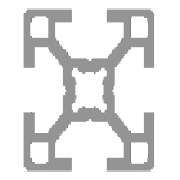
# Autodesk Inventor part: 30-3030
Saved by Autodesk Inventor 2021 (Build 250183000, 183)
## iProperties
_CCFamilyDisplayName: 30-3030
_FrameMemberDoc: Frame Member File
_Version: 25.0.0
_GetPNFromCC: 1
Created: 2020-11-08
Part Number: 30-3030
Material: Generic
Document SubType Name: Modeling
Designer: Wes
Manufacturer: 8020
Standards Organization: 8020 Metric
Language: en-US
Size Designation: 30-3030
Categories: <MemberInstance><Categories><Category DisplayName="Structural Shapes" InternalName="089c4875-fa83-4c05-b084-43b9cc11f5ed" Mnemonic="GRDR"><CategoryParameter DisplayName="Mass per Length Unit" InternalName="0bb95a10-148f-4027-a459-38d7b056702a" Mnemonic="shpmass"/><CategoryParameter DisplayName="Section Area" InternalName="1ff91680-64b0-4202-b9a3-7fd3f94bba3b" Mnemonic="secarea"/><CategoryParameter DisplayName="Radius of Gyration (x)" InternalName="25778675-03e9-40c1-b6a8-4a9ed693320d" Mnemonic="gyrradx"/><CategoryParameter DisplayName="Torsional Rigidity Modulus" InternalName="26c1ec35-5026-4c63-ad0a-751cf684a536" Mnemonic="torrigmod"/><CategoryParameter DisplayName="Distance of the Center of Gravity X-X" InternalName="26c9bdb8-9c79-4b4f-a92e-8e197583c9c4" Mnemonic="grcendistX"/><CategoryParameter DisplayName="Legacy Member ID" InternalName="340afe4f-75d7-48d3-ab7d-943f3c3da468" Mnemonic="LegacyMemberID"/><CategoryParameter DisplayName="Base Length" InternalName="42e34263-8f20-4d0e-ad48-bf1385b87c24" Mnemonic="shplen"/><CategoryParameter DisplayName="Moment of Inertia (y)" InternalName="4b9f58ea-bced-460e-81ea-3d29ca5a49e3" Mnemonic="inermomy"/><CategoryParameter DisplayName="Moment of Inertia (x)" InternalName="4cd780bc-73d7-43ac-917a-579e5cbd684d" Mnemonic="inermomx"/><CategoryParameter DisplayName="Custom Base Point" InternalName="4f1d1b73-316d-484b-a3df-9cbabb16eb77" Mnemonic="shpBasePoint"/><CategoryParameter DisplayName="Shape Height" InternalName="50274e7d-5ac0-4796-92cb-c59e54983c67" Mnemonic="shpheig"/><CategoryParameter DisplayName="Section Module (y)" InternalName="59eaa5e9-d227-48dc-b6c1-6920f96e0f95" Mnemonic="secmody"/><CategoryParameter DisplayName="Section Designation" InternalName="5a64d034-428d-49c8-ba32-7619764de20f" Mnemonic="shpdes"/><CategoryParameter DisplayName="Section Module (x)" InternalName="72cfad18-cf51-4ed4-aaa7-c6b224f8419f" Mnemonic="secmodx"/><CategoryParameter DisplayName="Torsional Section Modulus" InternalName="7c55a8dc-8844-49f9-a867-cc677b30ec9a" Mnemonic="torsecmod"/><CategoryParameter DisplayName="Shape Width" InternalName="7c717d54-a18f-4666-b4d4-573cce22c62c" Mnemonic="shpwdth"/><CategoryParameter DisplayName="Second Shape Thickness" InternalName="9251a8e1-85fd-4e47-af99-afdb762317d9" Mnemonic="shpthick2"/><CategoryParameter DisplayName="FG Authored" InternalName="9c666724-f362-4ea7-ac62-f6a007de5c69" Mnemonic="shpFGAuto"/><CategoryParameter DisplayName="Distance of the Center of Gravity Y-Y" InternalName="bcc4fb17-7af4-436a-8f8c-d0aa3b0248c5" Mnemonic="grcendistY"/><CategoryParameter DisplayName="Radius of Gyration (y)" InternalName="bfa18ebe-1636-4dbe-8d42-b263e0b73184" Mnemonic="gyrrady"/><CategoryParameter DisplayName="Shape Thickness" InternalName="d109cf76-8eb4-42fc-9800-4409734adc67" Mnemonic="shpthick"/><CategoryParameter DisplayName="Coefficient of Shear Displacement" InternalName="de4c90c6-aaa8-468f-a335-6737b311b5d3" Mnemonic="shdispc"/><Category DisplayName="Other" InternalName="f02205ff-2390-476f-921c-0b3185f88e84" Mnemonic="OTHSHP"><CategoryParameter DisplayName="Moment of Inertia (y)" InternalName="044c654e-f649-48ac-84cc-650a29ae31ca" Mnemonic="inermomy"/><CategoryParameter DisplayName="Shape Thickness" InternalName="12b1a788-9233-48fd-a933-2df8ff42b15f" Mnemonic="shpthick"/><CategoryParameter DisplayName="Mass per Length Unit" InternalName="2fd289d6-9394-4d2d-97e6-6659d7d4551d" Mnemonic="shpmass"/><CategoryParameter DisplayName="Radius of Gyration (y)" InternalName="743e1dfe-1bba-408b-b985-cf752b207386" Mnemonic="gyrrady"/><CategoryParameter DisplayName="Section Module (y)" InternalName="88b8bff9-a616-4028-93d5-ed4f79680d13" Mnemonic="secmody"/><CategoryParameter DisplayName="Section Area" InternalName="c46ecdf8-b6eb-4db9-8b25-30258930c1e3" Mnemonic="secarea"/><CategoryParameter DisplayName="Section Module (x)" InternalName="cac70804-9d39-43bb-be17-56ea1f39a6c2" Mnemonic="secmodx"/><CategoryParameter DisplayName="Moment of Inertia (x)" InternalName="ec6737bc-264f-43ed-b0bd-f6d410c2718d" Mnemonic="inermomx"/><CategoryParameter DisplayName="Radius of Gyration (x)" InternalName="ee72c61e-565e-4fd6-b448-66e1e1abcb7e" Mnemonic="gyrradx"/><Category DisplayName="8020" InternalName="79851eee-1260-43d5-80eb-d25638456875" Mnemonic="8020"/></Category></Category><Category DisplayName="DataType" InternalName="23b78d0f-2648-40c6-8793-ca6db495c9e8" Mnemonic="DATATYPE"><CategoryParameter DisplayName="DisplayName" InternalName="05415f3d-3907-474b-a020-eb9d644f4cf3" Mnemonic="DISPLAYNAME"/><CategoryParameter DisplayName="Standard" InternalName="0c0a119c-1e12-4c84-803f-101930972f5e" Mnemonic="STANDARD"/><CategoryParameter DisplayName="Description" InternalName="13903e3d-64b1-4950-80da-f627842ea37f" Mnemonic="DESCRIPTION"/><CategoryParameter DisplayName="Designation" InternalName="2675968c-4ce5-49e0-a4f5-552d29089031" Mnemonic="DESIGNATION"/><CategoryParameter DisplayName="Default Row" InternalName="2af9ec52-faaa-4026-b378-f9fa4afca842" Mnemonic="DEFAULTROW"/><CategoryParameter DisplayName="Folder Name" InternalName="3f06958e-8713-4116-9be7-ed6184ecc97b" Mnemonic="FOLDERNAME"/><CategoryParameter DisplayName="Revision Guid" InternalName="45a75005-10b1-4dfc-8d6d-dfe629f0b93c" Mnemonic="REVISIONGUID"/><CategoryParameter DisplayName="FileName" InternalName="8b46a4cc-9585-4fed-90c3-899f57e09a73" Mnemonic="FILENAME"/><CategoryParameter DisplayName="StdsOrg" InternalName="8f5914e1-4693-403f-8ab5-d37768198c9d" Mnemonic="STDSORG"/><CategoryParameter DisplayName="Family Version" InternalName="914462f6-6e19-4b14-ba84-155b9680b1d0" Mnemonic="FAMILYREVISION"/><CategoryParameter DisplayName="Standard Revision" InternalName="91d5a463-65c2-4fde-b823-3b7fea5e8e17" Mnemonic="STANDARDREVISION"/><CategoryParameter DisplayName="Member Revision" InternalName="a65d44b9-392f-4f4f-857b-e4b3d54996fe" Mnemonic="MEMBERREVISION"/><CategoryParameter DisplayName="ClipFormat" InternalName="bc51e27b-3422-4e78-93ef-cec197ddf230" Mnemonic="CLIPFORMAT"/><CategoryParameter DisplayName="Manufacturer" InternalName="cd6c7a72-a28a-4e50-99a9-2c7f4e13e5ad" Mnemonic="MANUFACTURER"/><CategoryParameter DisplayName="InternalName" InternalName="cf1d0246-76d9-4b4a-8305-fa0409afb5c1" Mnemonic="INTERNALNAME"/><CategoryParameter DisplayName="IsMetric" InternalName="e2385c5b-1ea4-4823-96a8-8de651266ec3" Mnemonic="ISMETRIC"/><Category DisplayName="Part" InternalName="c0e0b642-3bcb-4cc8-9e80-f96d35c4afa4" Mnemonic="PART"><CategoryParameter DisplayName="Part Number" InternalName="016b6077-bfbe-49bd-92c9-d8d59c39c941" Mnemonic="PARTNUMBER"/><CategoryParameter DisplayName="Stock Number" InternalName="4dba7c1c-e26c-444e-836c-b08b433409a8" Mnemonic="STOCKNUMBER"/><CategoryParameter DisplayName="Material Key" InternalName="5c9a8adb-dd2b-4535-b97f-0a94a95fe41f" Mnemonic="MATERIALKEY"/><CategoryParameter DisplayName="Material" InternalName="818a152a-d3c3-49ca-80ee-df7d91421b8e" Mnemonic="MATERIAL"/></Category></Category></Categories><FamilyTemplate Id="30-3030"><FamilyTemplateParameters><FamilyTemplateParameter ObjectType="kModelParameterObject" ValueType="xs:double" Id="12" ObjectReferenceKey="Length"/><FamilyTemplateParameter ObjectType="kPartComponentDefinitionObject" ValueType="xs:string" Id="23" SubObjectId="Material"/><FamilyTemplateParameter ObjectType="kPropertyObject" ValueType="xs:string" Id="26" ObjectReferenceKey="{32853F0F-3444-11d1-9E93-0060B03C1CA6}" SubObjectId="5"/><FamilyTemplateParameter ObjectType="kPropertyObject" ValueType="xs:string" Id="27" ObjectReferenceKey="{32853F0F-3444-11d1-9E93-0060B03C1CA6}" SubObjectId="52"/></FamilyTemplateParameters></FamilyTemplate><CategoryParameterMap><ParamToTemplateMap><ParamToTemplate CategoryParameter="//CategoryParameter[@InternalName='cf1d0246-76d9-4b4a-8305-fa0409afb5c1']" ConstantValue="0c7d1244-42aa-4641-8c1f-ef9d9099bed6"/><ParamToTemplate CategoryParameter="//CategoryParameter[@InternalName='45a75005-10b1-4dfc-8d6d-dfe629f0b93c']" ConstantValue="15f48215-b719-44ce-96ed-f2adf66c00d4"/><ParamToTemplate CategoryParameter="//CategoryParameter[@InternalName='3f06958e-8713-4116-9be7-ed6184ecc97b']" ConstantValue="30-3030"/><ParamToTemplate CategoryParameter="//CategoryParameter[@InternalName='8f5914e1-4693-403f-8ab5-d37768198c9d']" ConstantValue="8020 Metric"/><ParamToTemplate CategoryParameter="//CategoryParameter[@InternalName='0c0a119c-1e12-4c84-803f-101930972f5e']" TemplateParameter="18"/><ParamToTemplate CategoryParameter="//CategoryParameter[@InternalName='91d5a463-65c2-4fde-b823-3b7fea5e8e17']" TemplateParameter="19"/><ParamToTemplate CategoryParameter="//CategoryParameter[@InternalName='cd6c7a72-a28a-4e50-99a9-2c7f4e13e5ad']" ConstantValue="8020"/><ParamToTemplate CategoryParameter="//CategoryParameter[@InternalName='13903e3d-64b1-4950-80da-f627842ea37f']" TemplateParameter="22"/><ParamToTemplate CategoryParameter="//CategoryParameter[@InternalName='05415f3d-3907-474b-a020-eb9d644f4cf3']" ConstantValue="30-3030"/><ParamToTemplate CategoryParameter="//CategoryParameter[@InternalName='914462f6-6e19-4b14-ba84-155b9680b1d0']" ConstantValue="11"/><ParamToTemplate CategoryParameter="//CategoryParameter[@InternalName='bc51e27b-3422-4e78-93ef-cec197ddf230']" ConstantValue="CF_INVENTOR.STDPARTS"/><ParamToTemplate CategoryParameter="//CategoryParameter[@InternalName='e2385c5b-1ea4-4823-96a8-8de651266ec3']" ConstantValue="false"/><ParamToTemplate CategoryParameter="//CategoryParameter[@InternalName='2af9ec52-faaa-4026-b378-f9fa4afca842']" ConstantValue="1"/><ParamToTemplate CategoryParameter="//CategoryParameter[@InternalName='9c666724-f362-4ea7-ac62-f6a007de5c69']" ConstantValue="1"/><ParamToTemplate CategoryParameter="//CategoryParameter[@InternalName='8b46a4cc-9585-4fed-90c3-899f57e09a73']" ConstantValue="30-3030"/><ParamToTemplate CategoryParameter="//CategoryParameter[@InternalName='a65d44b9-392f-4f4f-857b-e4b3d54996fe']" ConstantValue="83db84f2-a349-434c-8932-27b256aad8d1"/><ParamToTemplate CategoryParameter="//CategoryParameter[@InternalName='a65d44b9-392f-4f4f-857b-e4b3d54996fe']" ConstantValue="83db84f2-a349-434c-8932-27b256aad8d1"/><ParamToTemplate CategoryParameter="//CategoryParameter[@InternalName='2675968c-4ce5-49e0-a4f5-552d29089031']" TemplateParameter="27"/><ParamToTemplate CategoryParameter="//CategoryParameter[@InternalName='42e34263-8f20-4d0e-ad48-bf1385b87c24']" TemplateParameter="12"/><ParamToTemplate CategoryParameter="//CategoryParameter[@InternalName='818a152a-d3c3-49ca-80ee-df7d91421b8e']" TemplateParameter="23"/><ParamToTemplate CategoryParameter="//CategoryParameter[@InternalName='016b6077-bfbe-49bd-92c9-d8d59c39c941']" TemplateParameter="26"/></ParamToTemplateMap></CategoryParameterMap></MemberInstance>
Density: 1 g/cm^3
Appearance: Default
IsCustomPart: 1
G_W: 1.181 in
G_H: 1.181 in
G_L: 34.016 in
+F1501FAD-5F95-4806-B732-5FE33EAD4360+CUTDETAIL1: Cut Angle 90.00 deg
Author: Wes
Autodesk Inventor part; units mm, degrees
sketch "30-3030" plane through (0, 0, 0) normal (0, 0, 1) x (1, 0, 0)
  arc A0 (-12.7342, 25.6778) -> (-12.3542, 25.2978) centre (-12.3542, 25.6778) ccw
  line L0 (-12.3542, 25.2978) -> (-8.9152, 25.2978)
  arc A1 (-8.9152, 25.2978) -> (-8.5342, 25.6788) centre (-8.9152, 25.6788) ccw
  line L1 (-8.5342, 25.6788) -> (-8.5342, 28.4978)
  arc A2 (-8.5342, 28.4978) -> (-9.5342, 29.4978) centre (-9.5342, 28.4978) ccw
  line L2 (-9.5342, 29.4978) -> (-12.3532, 29.4978)
  arc A3 (-12.3532, 29.4978) -> (-12.7342, 29.1168) centre (-12.3532, 29.1168) ccw
  line L3 (-12.7342, 29.1168) -> (-12.7342, 25.6778)
  arc A4 (-19.7608, 11.8179) -> (-18.2542, 13.3245) centre (-19.0919, 12.6556) ccw
  line L4 (-18.2542, 13.3245) -> (-19.036, 14.3036)
  arc A5 (-19.036, 14.3036) -> (-19.036, 17.2921) centre (-22.2341, 15.7978) ccw
  line L5 (-19.036, 17.2921) -> (-18.2542, 18.2712)
  arc A6 (-18.2542, 18.2712) -> (-19.7608, 19.7778) centre (-19.0919, 18.94) ccw
  line L6 (-19.7608, 19.7778) -> (-20.7399, 18.996)
  arc A7 (-20.7399, 18.996) -> (-23.7283, 18.996) centre (-22.2341, 15.7978) ccw
  line L7 (-23.7283, 18.996) -> (-24.7075, 19.7778)
  arc A8 (-24.7075, 19.7778) -> (-26.214, 18.2712) centre (-25.3763, 18.94) ccw
  line L8 (-26.214, 18.2712) -> (-25.4323, 17.2921)
  arc A9 (-25.4323, 17.2921) -> (-25.4323, 14.3036) centre (-22.2341, 15.7978) ccw
  line L9 (-25.4323, 14.3036) -> (-26.214, 13.3245)
  arc A10 (-26.214, 13.3245) -> (-24.7075, 11.8179) centre (-25.3763, 12.6556) ccw
  line L10 (-24.7075, 11.8179) -> (-23.7283, 12.5997)
  arc A11 (-23.7283, 12.5997) -> (-20.7399, 12.5997) centre (-22.2341, 15.7978) ccw
  line L11 (-20.7399, 12.5997) -> (-19.7608, 11.8179)
  arc A12 (-9.5342, 2.0979) -> (-8.5342, 3.0979) centre (-9.5342, 3.0979) ccw
  line L12 (-8.5342, 3.0979) -> (-8.5342, 5.9169)
  arc A13 (-8.5342, 5.9169) -> (-8.9152, 6.2979) centre (-8.9152, 5.9169) ccw
  line L13 (-8.9152, 6.2979) -> (-12.3542, 6.2979)
  arc A14 (-12.3542, 6.2979) -> (-12.7342, 5.9179) centre (-12.3542, 5.9179) ccw
  line L14 (-12.7342, 5.9179) -> (-12.7342, 2.4789)
  arc A15 (-12.7342, 2.4789) -> (-12.3532, 2.0979) centre (-12.3532, 2.4789) ccw
  line L15 (-12.3532, 2.0979) -> (-9.5342, 2.0979)
  line L16 (-7.7342, 11.7978) -> (-8.9916, 11.7978)
  arc A16 (-7.2342, 11.2978) -> (-7.7342, 11.7978) centre (-7.7342, 11.2978) ccw
  line L17 (-7.2342, 2.7979) -> (-7.2342, 11.2978)
  arc A17 (-9.2342, 0.7979) -> (-7.2342, 2.7979) centre (-9.2342, 2.7979) ccw
  line L18 (-17.7341, 0.7979) -> (-9.2342, 0.7979)
  arc A18 (-18.2341, 1.2979) -> (-17.7341, 0.7979) centre (-17.7341, 1.2979) ccw
  line L19 (-18.2341, 2.5554) -> (-18.2341, 1.2979)
  arc A19 (-17.7341, 3.0554) -> (-18.2341, 2.5554) centre (-17.7341, 2.5554) ccw
  line L20 (-14.5016, 3.0554) -> (-17.7341, 3.0554)
  arc A20 (-14.5016, 3.0554) -> (-13.9842, 3.555) centre (-14.4841, 3.555) ccw
  line L21 (-13.9842, 5.5376) -> (-13.9842, 3.555)
  arc A21 (-13.9842, 5.5376) -> (-14.1306, 5.8912) centre (-14.4841, 5.5376) ccw
  line L22 (-18.0561, 9.8167) -> (-14.1306, 5.8912)
  arc A22 (-18.0561, 9.8167) -> (-18.4097, 9.9632) centre (-18.4097, 9.4632) ccw
  line L23 (-21.2841, 9.9632) -> (-18.4097, 9.9632)
  line L24 (-22.2341, 10.4732) -> (-21.2841, 9.9632)
  line L25 (-23.1841, 9.9632) -> (-22.2341, 10.4732)
  line L26 (-26.0586, 9.9632) -> (-23.1841, 9.9632)
  arc A23 (-26.0586, 9.9632) -> (-26.4121, 9.8167) centre (-26.0586, 9.4632) ccw
  line L27 (-30.3376, 5.8912) -> (-26.4121, 9.8167)
  arc A24 (-30.3376, 5.8912) -> (-30.4841, 5.5376) centre (-29.9841, 5.5376) ccw
  line L28 (-30.4841, 3.555) -> (-30.4841, 5.5376)
  arc A25 (-30.4841, 3.555) -> (-29.9666, 3.0554) centre (-29.9841, 3.555) ccw
  line L29 (-26.7341, 3.0554) -> (-29.9666, 3.0554)
  arc A26 (-26.2341, 2.5554) -> (-26.7341, 3.0554) centre (-26.7341, 2.5554) ccw
  line L30 (-26.2341, 1.2979) -> (-26.2341, 2.5554)
  arc A27 (-26.7341, 0.7979) -> (-26.2341, 1.2979) centre (-26.7341, 1.2979) ccw
  line L31 (-35.2341, 0.7979) -> (-26.7341, 0.7979)
  arc A28 (-37.2341, 2.7979) -> (-35.2341, 0.7979) centre (-35.2341, 2.7979) ccw
  line L32 (-37.2341, 11.2978) -> (-37.2341, 2.7979)
  arc A29 (-36.7341, 11.7978) -> (-37.2341, 11.2978) centre (-36.7341, 11.2978) ccw
  line L33 (-35.4766, 11.7978) -> (-36.7341, 11.7978)
  arc A30 (-34.9766, 11.2978) -> (-35.4766, 11.7978) centre (-35.4766, 11.2978) ccw
  line L34 (-34.9766, 8.0653) -> (-34.9766, 11.2978)
  arc A31 (-34.9766, 8.0653) -> (-34.4769, 7.5479) centre (-34.4769, 8.0479) ccw
  line L35 (-32.4943, 7.5479) -> (-34.4769, 7.5479)
  arc A32 (-32.4943, 7.5479) -> (-32.1408, 7.6943) centre (-32.4943, 8.0479) ccw
  line L36 (-28.2152, 11.6198) -> (-32.1408, 7.6943)
  arc A33 (-28.2152, 11.6198) -> (-28.0688, 11.9734) centre (-28.5688, 11.9734) ccw
  line L37 (-28.0688, 14.7853) -> (-28.0688, 11.9734)
  line L38 (-27.5588, 15.7353) -> (-28.0688, 14.7853)
  line L39 (-28.0688, 16.6853) -> (-27.5588, 15.7353)
  line L40 (-28.0688, 19.6223) -> (-28.0688, 16.6853)
  arc A34 (-28.0688, 19.6223) -> (-28.2152, 19.9758) centre (-28.5688, 19.6223) ccw
  line L41 (-32.1408, 23.9013) -> (-28.2152, 19.9758)
  arc A35 (-32.1408, 23.9013) -> (-32.4943, 24.0478) centre (-32.4943, 23.5478) ccw
  line L42 (-34.4769, 24.0478) -> (-32.4943, 24.0478)
  arc A36 (-34.4769, 24.0478) -> (-34.9766, 23.5303) centre (-34.4769, 23.5478) ccw
  line L43 (-34.9766, 20.2978) -> (-34.9766, 23.5303)
  arc A37 (-35.4766, 19.7978) -> (-34.9766, 20.2978) centre (-35.4766, 20.2978) ccw
  line L44 (-36.7341, 19.7978) -> (-35.4766, 19.7978)
  arc A38 (-37.2341, 20.2978) -> (-36.7341, 19.7978) centre (-36.7341, 20.2978) ccw
  line L45 (-37.2341, 28.7978) -> (-37.2341, 20.2978)
  arc A39 (-35.2341, 30.7978) -> (-37.2341, 28.7978) centre (-35.2341, 28.7978) ccw
  line L46 (-26.7341, 30.7978) -> (-35.2341, 30.7978)
  arc A40 (-26.2341, 30.2978) -> (-26.7341, 30.7978) centre (-26.7341, 30.2978) ccw
  line L47 (-26.2341, 29.0403) -> (-26.2341, 30.2978)
  arc A41 (-26.7341, 28.5403) -> (-26.2341, 29.0403) centre (-26.7341, 29.0403) ccw
  line L48 (-29.9666, 28.5403) -> (-26.7341, 28.5403)
  arc A42 (-29.9666, 28.5403) -> (-30.4841, 28.0406) centre (-29.9841, 28.0406) ccw
  line L49 (-30.4841, 26.058) -> (-30.4841, 28.0406)
  arc A43 (-30.4841, 26.058) -> (-30.3376, 25.7045) centre (-29.9841, 26.058) ccw
  line L50 (-26.4121, 21.7789) -> (-30.3376, 25.7045)
  arc A44 (-26.4121, 21.7789) -> (-26.0586, 21.6325) centre (-26.0586, 22.1325) ccw
  line L51 (-23.1841, 21.6325) -> (-26.0586, 21.6325)
  line L52 (-22.2341, 21.1225) -> (-23.1841, 21.6325)
  line L53 (-21.2841, 21.6325) -> (-22.2341, 21.1225)
  line L54 (-18.4097, 21.6325) -> (-21.2841, 21.6325)
  arc A45 (-18.4097, 21.6325) -> (-18.0561, 21.7789) centre (-18.4097, 22.1325) ccw
  line L55 (-14.1306, 25.7045) -> (-18.0561, 21.7789)
  arc A46 (-14.1306, 25.7045) -> (-13.9842, 26.058) centre (-14.4841, 26.058) ccw
  line L56 (-13.9842, 28.0406) -> (-13.9842, 26.058)
  arc A47 (-13.9842, 28.0406) -> (-14.5016, 28.5403) centre (-14.4841, 28.0406) ccw
  line L57 (-17.7341, 28.5403) -> (-14.5016, 28.5403)
  arc A48 (-18.2341, 29.0403) -> (-17.7341, 28.5403) centre (-17.7341, 29.0403) ccw
  line L58 (-18.2341, 30.2978) -> (-18.2341, 29.0403)
  arc A49 (-17.7341, 30.7978) -> (-18.2341, 30.2978) centre (-17.7341, 30.2978) ccw
  line L59 (-9.2342, 30.7978) -> (-17.7341, 30.7978)
  arc A50 (-7.2342, 28.7978) -> (-9.2342, 30.7978) centre (-9.2342, 28.7978) ccw
  line L60 (-7.2342, 20.2978) -> (-7.2342, 28.7978)
  arc A51 (-7.7342, 19.7978) -> (-7.2342, 20.2978) centre (-7.7342, 20.2978) ccw
  line L61 (-8.9916, 19.7978) -> (-7.7342, 19.7978)
  arc A52 (-9.4916, 20.2978) -> (-8.9916, 19.7978) centre (-8.9916, 20.2978) ccw
  line L62 (-9.4916, 23.5303) -> (-9.4916, 20.2978)
  arc A53 (-9.4916, 23.5303) -> (-9.9913, 24.0478) centre (-9.9913, 23.5478) ccw
  line L63 (-11.9739, 24.0478) -> (-9.9913, 24.0478)
  arc A54 (-11.9739, 24.0478) -> (-12.3275, 23.9013) centre (-11.9739, 23.5478) ccw
  line L64 (-16.253, 19.9758) -> (-12.3275, 23.9013)
  arc A55 (-16.253, 19.9758) -> (-16.3994, 19.6223) centre (-15.8994, 19.6223) ccw
  line L65 (-16.3994, 16.6853) -> (-16.3994, 19.6223)
  line L66 (-16.9094, 15.7353) -> (-16.3994, 16.6853)
  line L67 (-16.3994, 14.7853) -> (-16.9094, 15.7353)
  line L68 (-16.3994, 11.9734) -> (-16.3994, 14.7853)
  arc A56 (-16.3994, 11.9734) -> (-16.253, 11.6198) centre (-15.8994, 11.9734) ccw
  line L69 (-12.3275, 7.6943) -> (-16.253, 11.6198)
  arc A57 (-12.3275, 7.6943) -> (-11.9739, 7.5479) centre (-11.9739, 8.0479) ccw
  line L70 (-9.9913, 7.5479) -> (-11.9739, 7.5479)
  arc A58 (-9.9913, 7.5479) -> (-9.4916, 8.0653) centre (-9.9913, 8.0479) ccw
  line L71 (-9.4916, 11.2978) -> (-9.4916, 8.0653)
  arc A59 (-8.9916, 11.7978) -> (-9.4916, 11.2978) centre (-8.9916, 11.2978) ccw
  arc A60 (-35.9341, 3.0979) -> (-34.9341, 2.0979) centre (-34.9341, 3.0979) ccw
  line L72 (-34.9341, 2.0979) -> (-32.1151, 2.0979)
  arc A61 (-32.1151, 2.0979) -> (-31.7341, 2.4789) centre (-32.1151, 2.4789) ccw
  line L73 (-31.7341, 2.4789) -> (-31.7341, 5.9179)
  arc A62 (-31.7341, 5.9179) -> (-32.1141, 6.2979) centre (-32.1141, 5.9179) ccw
  line L74 (-32.1141, 6.2979) -> (-35.5531, 6.2979)
  arc A63 (-35.5531, 6.2979) -> (-35.9341, 5.9169) centre (-35.5531, 5.9169) ccw
  line L75 (-35.9341, 5.9169) -> (-35.9341, 3.0979)
  arc A64 (-34.9341, 29.4978) -> (-35.9341, 28.4978) centre (-34.9341, 28.4978) ccw
  line L76 (-35.9341, 28.4978) -> (-35.9341, 25.6788)
  arc A65 (-35.9341, 25.6788) -> (-35.5531, 25.2978) centre (-35.5531, 25.6788) ccw
  line L77 (-35.5531, 25.2978) -> (-32.1141, 25.2978)
  arc A66 (-32.1141, 25.2978) -> (-31.7341, 25.6778) centre (-32.1141, 25.6778) ccw
  line L78 (-31.7341, 25.6778) -> (-31.7341, 29.1168)
  arc A67 (-31.7341, 29.1168) -> (-32.1151, 29.4978) centre (-32.1151, 29.1168) ccw
  line L79 (-32.1151, 29.4978) -> (-34.9341, 29.4978)
ref_plane "Start Plane" through (0, 0, -29.9999) normal (0, 0, 1) x (1, 0, 0)
ref_plane "End Plane" through (0, 0, 834) normal (0, 0, 1) x (1, 0, 0)
sketch "Sketch" plane through (0, 0, 0) normal (0, 0, 1) x (1, 0, 0)
  arc A0 (9.5, 9.88) -> (9.88, 9.5) centre (9.88, 9.88) ccw
  line L0 (9.88, 9.5) -> (13.3189, 9.5)
  arc A1 (13.3189, 9.5) -> (13.6999, 9.881) centre (13.3189, 9.881) ccw
  line L1 (13.6999, 9.881) -> (13.6999, 12.6999)
  arc A2 (13.6999, 12.6999) -> (12.6999, 13.6999) centre (12.6999, 12.6999) ccw
  line L2 (12.6999, 13.6999) -> (9.881, 13.6999)
  arc A3 (9.881, 13.6999) -> (9.5, 13.3189) centre (9.881, 13.3189) ccw
  line L3 (9.5, 13.3189) -> (9.5, 9.88)
  arc A4 (2.4733, -3.9799) -> (3.9799, -2.4733) centre (3.1422, -3.1422) ccw
  line L4 (3.9799, -2.4733) -> (3.1981, -1.4942)
  arc A5 (3.1981, -1.4942) -> (3.1981, 1.4942) centre (0, 0) ccw
  line L5 (3.1981, 1.4942) -> (3.9799, 2.4733)
  arc A6 (3.9799, 2.4733) -> (2.4733, 3.9799) centre (3.1422, 3.1422) ccw
  line L6 (2.4733, 3.9799) -> (1.4942, 3.1981)
  arc A7 (1.4942, 3.1981) -> (-1.4942, 3.1981) centre (0, 0) ccw
  line L7 (-1.4942, 3.1981) -> (-2.4733, 3.9799)
  arc A8 (-2.4733, 3.9799) -> (-3.9799, 2.4733) centre (-3.1422, 3.1422) ccw
  line L8 (-3.9799, 2.4733) -> (-3.1981, 1.4942)
  arc A9 (-3.1981, 1.4942) -> (-3.1981, -1.4942) centre (0, 0) ccw
  line L9 (-3.1981, -1.4942) -> (-3.9799, -2.4733)
  arc A10 (-3.9799, -2.4733) -> (-2.4733, -3.9799) centre (-3.1422, -3.1422) ccw
  line L10 (-2.4733, -3.9799) -> (-1.4942, -3.1981)
  arc A11 (-1.4942, -3.1981) -> (1.4942, -3.1981) centre (0, 0) ccw
  line L11 (1.4942, -3.1981) -> (2.4733, -3.9799)
  arc A12 (12.6999, -13.6999) -> (13.6999, -12.6999) centre (12.6999, -12.6999) ccw
  line L12 (13.6999, -12.6999) -> (13.6999, -9.881)
  arc A13 (13.6999, -9.881) -> (13.3189, -9.5) centre (13.3189, -9.881) ccw
  line L13 (13.3189, -9.5) -> (9.88, -9.5)
  arc A14 (9.88, -9.5) -> (9.5, -9.88) centre (9.88, -9.88) ccw
  line L14 (9.5, -9.88) -> (9.5, -13.3189)
  arc A15 (9.5, -13.3189) -> (9.881, -13.6999) centre (9.881, -13.3189) ccw
  line L15 (9.881, -13.6999) -> (12.6999, -13.6999)
  line L16 (14.4999, -4) -> (13.2425, -4)
  arc A16 (14.9999, -4.5) -> (14.4999, -4) centre (14.4999, -4.5) ccw
  line L17 (14.9999, -12.9999) -> (14.9999, -4.5)
  arc A17 (12.9999, -14.9999) -> (14.9999, -12.9999) centre (12.9999, -12.9999) ccw
  line L18 (4.5, -14.9999) -> (12.9999, -14.9999)
  arc A18 (4, -14.4999) -> (4.5, -14.9999) centre (4.5, -14.4999) ccw
  line L19 (4, -13.2425) -> (4, -14.4999)
  arc A19 (4.5, -12.7425) -> (4, -13.2425) centre (4.5, -13.2425) ccw
  line L20 (7.7325, -12.7425) -> (4.5, -12.7425)
  arc A20 (7.7325, -12.7425) -> (8.25, -12.2428) centre (7.75, -12.2428) ccw
  line L21 (8.25, -10.2602) -> (8.25, -12.2428)
  arc A21 (8.25, -10.2602) -> (8.1035, -9.9066) centre (7.75, -10.2602) ccw
  line L22 (4.178, -5.9811) -> (8.1035, -9.9066)
  arc A22 (4.178, -5.9811) -> (3.8245, -5.8347) centre (3.8245, -6.3347) ccw
  line L23 (0.95, -5.8347) -> (3.8245, -5.8347)
  line L24 (0, -5.3247) -> (0.95, -5.8347)
  line L25 (-0.95, -5.8347) -> (0, -5.3247)
  line L26 (-3.8245, -5.8347) -> (-0.95, -5.8347)
  arc A23 (-3.8245, -5.8347) -> (-4.178, -5.9811) centre (-3.8245, -6.3347) ccw
  line L27 (-8.1035, -9.9066) -> (-4.178, -5.9811)
  arc A24 (-8.1035, -9.9066) -> (-8.25, -10.2602) centre (-7.75, -10.2602) ccw
  line L28 (-8.25, -12.2428) -> (-8.25, -10.2602)
  arc A25 (-8.25, -12.2428) -> (-7.7325, -12.7425) centre (-7.75, -12.2428) ccw
  line L29 (-4.5, -12.7425) -> (-7.7325, -12.7425)
  arc A26 (-4, -13.2425) -> (-4.5, -12.7425) centre (-4.5, -13.2425) ccw
  line L30 (-4, -14.4999) -> (-4, -13.2425)
  arc A27 (-4.5, -14.9999) -> (-4, -14.4999) centre (-4.5, -14.4999) ccw
  line L31 (-12.9999, -14.9999) -> (-4.5, -14.9999)
  arc A28 (-14.9999, -12.9999) -> (-12.9999, -14.9999) centre (-12.9999, -12.9999) ccw
  line L32 (-14.9999, -4.5) -> (-14.9999, -12.9999)
  arc A29 (-14.4999, -4) -> (-14.9999, -4.5) centre (-14.4999, -4.5) ccw
  line L33 (-13.2425, -4) -> (-14.4999, -4)
  arc A30 (-12.7425, -4.5) -> (-13.2425, -4) centre (-13.2425, -4.5) ccw
  line L34 (-12.7425, -7.7325) -> (-12.7425, -4.5)
  arc A31 (-12.7425, -7.7325) -> (-12.2428, -8.25) centre (-12.2428, -7.75) ccw
  line L35 (-10.2602, -8.25) -> (-12.2428, -8.25)
  arc A32 (-10.2602, -8.25) -> (-9.9066, -8.1035) centre (-10.2602, -7.75) ccw
  line L36 (-5.9811, -4.178) -> (-9.9066, -8.1035)
  arc A33 (-5.9811, -4.178) -> (-5.8347, -3.8245) centre (-6.3347, -3.8245) ccw
  line L37 (-5.8347, -1.0125) -> (-5.8347, -3.8245)
  line L38 (-5.3247, -0.0625) -> (-5.8347, -1.0125)
  line L39 (-5.8347, 0.8875) -> (-5.3247, -0.0625)
  line L40 (-5.8347, 3.8245) -> (-5.8347, 0.8875)
  arc A34 (-5.8347, 3.8245) -> (-5.9811, 4.178) centre (-6.3347, 3.8245) ccw
  line L41 (-9.9066, 8.1035) -> (-5.9811, 4.178)
  arc A35 (-9.9066, 8.1035) -> (-10.2602, 8.25) centre (-10.2602, 7.75) ccw
  line L42 (-12.2428, 8.25) -> (-10.2602, 8.25)
  arc A36 (-12.2428, 8.25) -> (-12.7425, 7.7325) centre (-12.2428, 7.75) ccw
  line L43 (-12.7425, 4.5) -> (-12.7425, 7.7325)
  arc A37 (-13.2425, 4) -> (-12.7425, 4.5) centre (-13.2425, 4.5) ccw
  line L44 (-14.4999, 4) -> (-13.2425, 4)
  arc A38 (-14.9999, 4.5) -> (-14.4999, 4) centre (-14.4999, 4.5) ccw
  line L45 (-14.9999, 12.9999) -> (-14.9999, 4.5)
  arc A39 (-12.9999, 14.9999) -> (-14.9999, 12.9999) centre (-12.9999, 12.9999) ccw
  line L46 (-4.5, 14.9999) -> (-12.9999, 14.9999)
  arc A40 (-4, 14.4999) -> (-4.5, 14.9999) centre (-4.5, 14.4999) ccw
  line L47 (-4, 13.2425) -> (-4, 14.4999)
  arc A41 (-4.5, 12.7425) -> (-4, 13.2425) centre (-4.5, 13.2425) ccw
  line L48 (-7.7325, 12.7425) -> (-4.5, 12.7425)
  arc A42 (-7.7325, 12.7425) -> (-8.25, 12.2428) centre (-7.75, 12.2428) ccw
  line L49 (-8.25, 10.2602) -> (-8.25, 12.2428)
  arc A43 (-8.25, 10.2602) -> (-8.1035, 9.9066) centre (-7.75, 10.2602) ccw
  line L50 (-4.178, 5.9811) -> (-8.1035, 9.9066)
  arc A44 (-4.178, 5.9811) -> (-3.8245, 5.8347) centre (-3.8245, 6.3347) ccw
  line L51 (-0.95, 5.8347) -> (-3.8245, 5.8347)
  line L52 (0, 5.3247) -> (-0.95, 5.8347)
  line L53 (0.95, 5.8347) -> (0, 5.3247)
  line L54 (3.8245, 5.8347) -> (0.95, 5.8347)
  arc A45 (3.8245, 5.8347) -> (4.178, 5.9811) centre (3.8245, 6.3347) ccw
  line L55 (8.1035, 9.9066) -> (4.178, 5.9811)
  arc A46 (8.1035, 9.9066) -> (8.25, 10.2602) centre (7.75, 10.2602) ccw
  line L56 (8.25, 12.2428) -> (8.25, 10.2602)
  arc A47 (8.25, 12.2428) -> (7.7325, 12.7425) centre (7.75, 12.2428) ccw
  line L57 (4.5, 12.7425) -> (7.7325, 12.7425)
  arc A48 (4, 13.2425) -> (4.5, 12.7425) centre (4.5, 13.2425) ccw
  line L58 (4, 14.4999) -> (4, 13.2425)
  arc A49 (4.5, 14.9999) -> (4, 14.4999) centre (4.5, 14.4999) ccw
  line L59 (12.9999, 14.9999) -> (4.5, 14.9999)
  arc A50 (14.9999, 12.9999) -> (12.9999, 14.9999) centre (12.9999, 12.9999) ccw
  line L60 (14.9999, 4.5) -> (14.9999, 12.9999)
  arc A51 (14.4999, 4) -> (14.9999, 4.5) centre (14.4999, 4.5) ccw
  line L61 (13.2425, 4) -> (14.4999, 4)
  arc A52 (12.7425, 4.5) -> (13.2425, 4) centre (13.2425, 4.5) ccw
  line L62 (12.7425, 7.7325) -> (12.7425, 4.5)
  arc A53 (12.7425, 7.7325) -> (12.2428, 8.25) centre (12.2428, 7.75) ccw
  line L63 (10.2602, 8.25) -> (12.2428, 8.25)
  arc A54 (10.2602, 8.25) -> (9.9066, 8.1035) centre (10.2602, 7.75) ccw
  line L64 (5.9811, 4.178) -> (9.9066, 8.1035)
  arc A55 (5.9811, 4.178) -> (5.8347, 3.8245) centre (6.3347, 3.8245) ccw
  line L65 (5.8347, 0.8875) -> (5.8347, 3.8245)
  line L66 (5.3247, -0.0625) -> (5.8347, 0.8875)
  line L67 (5.8347, -1.0125) -> (5.3247, -0.0625)
  line L68 (5.8347, -3.8245) -> (5.8347, -1.0125)
  arc A56 (5.8347, -3.8245) -> (5.9811, -4.178) centre (6.3347, -3.8245) ccw
  line L69 (9.9066, -8.1035) -> (5.9811, -4.178)
  arc A57 (9.9066, -8.1035) -> (10.2602, -8.25) centre (10.2602, -7.75) ccw
  line L70 (12.2428, -8.25) -> (10.2602, -8.25)
  arc A58 (12.2428, -8.25) -> (12.7425, -7.7325) centre (12.2428, -7.75) ccw
  line L71 (12.7425, -4.5) -> (12.7425, -7.7325)
  arc A59 (13.2425, -4) -> (12.7425, -4.5) centre (13.2425, -4.5) ccw
  arc A60 (-13.6999, -12.6999) -> (-12.6999, -13.6999) centre (-12.6999, -12.6999) ccw
  line L72 (-12.6999, -13.6999) -> (-9.881, -13.6999)
  arc A61 (-9.881, -13.6999) -> (-9.5, -13.3189) centre (-9.881, -13.3189) ccw
  line L73 (-9.5, -13.3189) -> (-9.5, -9.88)
  arc A62 (-9.5, -9.88) -> (-9.88, -9.5) centre (-9.88, -9.88) ccw
  line L74 (-9.88, -9.5) -> (-13.3189, -9.5)
  arc A63 (-13.3189, -9.5) -> (-13.6999, -9.881) centre (-13.3189, -9.881) ccw
  line L75 (-13.6999, -9.881) -> (-13.6999, -12.6999)
  arc A64 (-12.6999, 13.6999) -> (-13.6999, 12.6999) centre (-12.6999, 12.6999) ccw
  line L76 (-13.6999, 12.6999) -> (-13.6999, 9.881)
  arc A65 (-13.6999, 9.881) -> (-13.3189, 9.5) centre (-13.3189, 9.881) ccw
  line L77 (-13.3189, 9.5) -> (-9.88, 9.5)
  arc A66 (-9.88, 9.5) -> (-9.5, 9.88) centre (-9.88, 9.88) ccw
  line L78 (-9.5, 9.88) -> (-9.5, 13.3189)
  arc A67 (-9.5, 13.3189) -> (-9.881, 13.6999) centre (-9.881, 13.3189) ccw
  line L79 (-9.881, 13.6999) -> (-12.6999, 13.6999)
  point P0 (0, 0)
  constraints: 1 other
extrude "Body" add sketch "Sketch" along normal up to surface (863.9999 mm away) from surface at -29.9999
sketch "Sketch2" plane through (0, 0, 0) normal (0, 0, 1) x (1, 0, 0)
  line L0 (0, 0) -> (10, 0)
ref_plane "Work Plane3" through (0, 0, 0) normal (0, -1, 0) x (1, 0, 0)
sketch "Sketch3" plane through (0, 0, 0) normal (0, -1, 0) x (1, 0, 0)
  line L0 (-2, -29.9999) -> (12, -29.9999)
  line L1 (-2, 834) -> (12, 834)
  dimension "d7" = 863.9999
  measures "d7" distance between parallel lines of L0 L1
ref_plane "Work Plane5" through (-822.0001, -13, -29.9999) normal (0, 0, -1) x (-1, 0, 0)
split "Split2" plane through (-822.0001, -13, -29.9999) removes the side toward (0, 0, -1)
equation "\"G_OFFSET_START\" = 29.99994"
equation "\"G_OFFSET_END\" = 0"
equation "\"d2\" = -G_OFFSET_START"
equation "\"d3\" = Length + G_OFFSET_END"
equation "\"G_L\" = d7"
equation "\"Length\" = 834"
body "Solid1"
